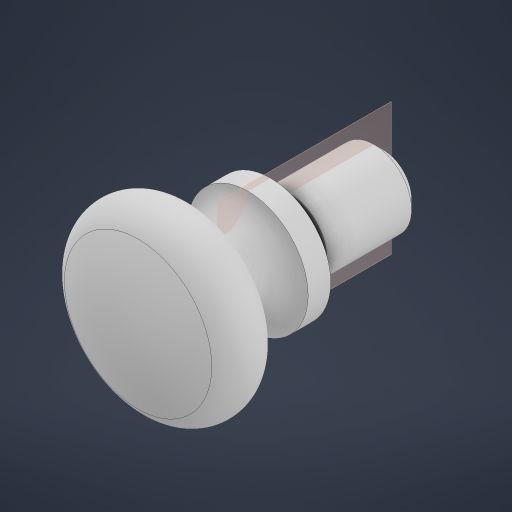
# Autodesk Inventor part: PartA
Saved by Autodesk Inventor 2024.3 (Build 283343000, 343)
## iProperties
Created: 2025-07-11
Part Number: PartA
Material: Generic
Document SubType Name: Modeling
Designer: LeoFB
Density: 1 g/cm^3
Appearance: Default
Author: LeoFB
Autodesk Inventor part; units mm, degrees
ref_plane "YZ Plane" through (0, 0, 0) normal (1, 0, 0) x (0, 1, 0)
ref_plane "XZ Plane" through (0, 0, 0) normal (0, 1, 0) x (-1, 0, 0)
ref_plane "XY Plane" through (0, 0, 0) normal (0, 0, 1) x (1, 0, 0)
sketch "Sketch1" plane through (0, 0, 0) normal (0, 0, 1) x (1, 0, 0)
  circle A0 centre (0, 0) radius 20
  dimension "d0" = 40
  constraints: 1 centre point, 1 coincident
  measures "d0" diameter of A0
extrude "Extrusion1" add sketch "Sketch1" along normal mid plane 50
chamfer "Chamfer1" distance 5 angle 45 1 edges at (-20, 0, -25)
ref_plane "Work Plane1" through (0, 0, 35) normal (0, 0, 1) x (1, 0, 0)
sketch "Sketch2" plane through (0, 0, 25) normal (0, 0, 1) x (1, 0, 0)
  point P0 (0, 0)
sketch "Sketch3" plane through (0, 0, 35) normal (0, 0, 1) x (1, 0, 0)
  circle A0 centre (0, 0) radius 32
  dimension "d7" = 64
  constraints: 1 centre point, 1 coincident
  measures "d7" diameter of A0
extrude "Extrusion2" add sketch "Sketch3" along normal blind 12
ref_plane "Work Plane2" through (0, -25, 47) normal (1, 0, 0) x (0, 0, -1)
sketch "Sketch5" plane through (0, -25, 47) normal (1, 0, 0) x (0, 0, -1)
  line L0 (22, 45) -> (22, 5) projected
  line L1 (22, 45) -> (32, 45) construction
  arc A0 (12, 45) -> (22, 45) centre (17, 45) ccw
  line L2 (22, 25) -> (12, 25)
  line L3 (12, 57) -> (12, -7) projected
  line L4 (12, 25) -> (12, 45)
  line L5 (22, 25) -> (22, 45)
  point P0 (47, 25)
  constraints: 8 end point, 2 midpoint, 2 point on circle, 1 centre point, 1 collinear, 1 horizontal, 1 point on line
revolve "Revolution1" add sketch "Sketch5" angle 360 about axis through (0, 0, 25) along (0, 0, 1)
sketch "Sketch6" plane through (0, -25, 47) normal (1, 0, 0) x (0, 0, -1)
  line L0 (12, 57) -> (0, 57) projected
  arc A0 (-28, 57) -> (0, 57) centre (-14, 57) ccw
  line L1 (0, 57) -> (0, -7) projected
  line L2 (0, 25) -> (28, 25) construction
  line L3 (0, 57) -> (0, 25)
  arc A1 (-28, 57) -> (-58.3251, 64.1269) centre (-44, 57) ccw
  line L4 (-29.6753, 49.8723) -> (7.9318, 49.8723) construction
  arc A2 (-58.3251, 64.1269) -> (-67.5205, 25) centre (20.32, 25) ccw
  line L5 (0, 25) -> (-67.5205, 25)
  point P0 (47, 25)
  dimension "d25" = 32
  constraints: 8 end point, 7 point on circle, 3 centre point, 3 horizontal, 2 point on line, 1 midpoint
  measures "d25" diameter of A1
revolve "Revolution2" add sketch "Sketch6" angle 360 about axis through (0, 0, 47) along (0, 0, 1)
body "Solid1"
